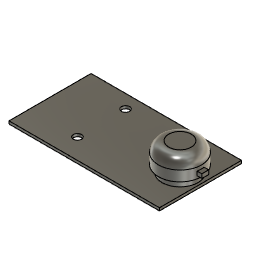
Controller Top (Autodesk Fusion 360 design; units mm, degrees)
Autodesk Fusion 360 part; units mm, degrees
note: some values were not read from the file. Chosen so that the rebuilt part matches the saved one: which face or edge a step refers to.
sketch "Sketch1" plane through (0, 0, 0) normal (0, 0, 1) x (1, 0, 0)
  line L0 (65, -25) -> (-45, -25)
  line L1 (-45, -25) -> (-45, 35)
  line L2 (-45, 35) -> (65, 35)
  line L3 (65, 35) -> (65, -25)
  constraint horizontal L0
  constraint vertical L1
  constraint horizontal L2
  constraint vertical L3
extrude "Extrude1" add sketch "Sketch1" along normal blind 3 and the other way blind -5 makes body 1
sketch "Sketch2" plane through (0, 0, 5) normal (0, 0, 1) x (-1, 0, 0)
  line L0 (-65, -35) -> (45, -35)
  line L1 (45, -35) -> (45, 25)
  line L2 (45, 25) -> (-65, 25)
  line L3 (-65, 25) -> (-65, -35)
  circle A0 centre (-50, -5) radius 13.1556
extrude "Extrude2" add sketch "Sketch2" along normal blind 5 contours A0 bodies 1
sketch "Sketch3" plane through (0, 0, 10) normal (0, 0, 1) x (-1, 0, 0)
  circle A0 centre (-50, -5) radius 13.1556
  circle A1 centre (-50, -5) radius 15.758
  constraint concentric A0 A1
extrude "Extrude3" add sketch "Sketch3" along normal blind 15 contours A0 | A1 bodies 1
fillet "Fillet1" radius 7.5 1 edges at (65.758, 5, 25) on bodies 1
sketch "Sketch4" plane through (0, 0, 0) normal (1, 0, 0) x (0, 1, 0)
  line L0 (2, 15) -> (7, 15)
  line L1 (7, 15) -> (7, 12)
  line L2 (7, 12) -> (2, 12)
  line L3 (2, 12) -> (2, 15)
  constraint horizontal L0
  constraint vertical L1
  constraint horizontal L2
  constraint vertical L3
extrude "Extrude4" add sketch "Sketch4" along normal blind 6 separate body makes body 2
move_body "MoveFace1" bodies 2 to x (1, 0, 0) y (0, 1, 0) z (0, 0, 1) at (63, 0, 0) on bodies 2
combine "Combine1" operation add target body 1 tool bodies 2
hole "Hole1" at (-9.8493, -10.1026, 5) direction (0, 0, -1) diameter 6 depth 5 tip angle 118 bodies 1
hole "Hole2" at (-9.9241, 25.1282, 5) direction (0, 0, -1) diameter 6 depth 4 tip angle 118 bodies 1
